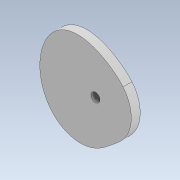
# Autodesk Inventor part: 凸輪
Saved by Autodesk Inventor 2022 (Build 260153000, 153)
## iProperties
Created: 2023-05-12
Part Number: 凸輪
Material: 一般
Document SubType Name: Modeling
Designer: JOU
Density: 1 g/cm^3
Appearance: 預設
Author: JOU
Autodesk Inventor part; units mm, degrees
ref_plane "YZ Plane" through (0, 0, 0) normal (1, 0, 0) x (0, 1, 0)
ref_plane "XZ Plane" through (0, 0, 0) normal (0, 1, 0) x (-1, 0, 0)
ref_plane "XY Plane" through (0, 0, 0) normal (0, 0, 1) x (1, 0, 0)
sketch "草圖1" plane through (0, 0, 0) normal (0, 0, 1) x (1, 0, 0)
  spline S0 degree 3 poles (30.808, 25.5122) (30.6572, 25.6926) (30.3546, 26.0547) (29.8877, 26.5903) (29.4098, 27.1227) (28.9202, 27.6516) (28.4194, 28.177) (27.9076, 28.6992) (27.3849, 29.2182) (26.8516, 29.7342) (26.3079, 30.2472) (25.754, 30.7574) (25.1901, 31.2648) (24.6164, 31.7697) (24.033, 32.2719) (23.44, 32.7717) (22.8377, 33.2691) (22.2261, 33.7641) (21.6054, 34.2567) (20.9756, 34.7471) (20.3368, 35.2351) (19.6892, 35.7208) (19.0327, 36.2041) (18.3675, 36.6849) (17.6935, 37.1633) (17.0109, 37.639) (16.3195, 38.112) (15.6195, 38.5821) (14.9108, 39.0491) (14.1934, 39.5129) (13.4673, 39.9733) (12.7325, 40.4299) (11.9891, 40.8827) (11.2369, 41.3311) (10.4759, 41.775) (9.7063, 42.2141) (8.9279, 42.6479) (8.1408, 43.0762) (7.3451, 43.4985) (6.5407, 43.9144) (5.7276, 44.3234) (4.9061, 44.7252) (4.0761, 45.1193) (3.2377, 45.5052) (2.3911, 45.8823) (1.5363, 46.2503) (0.6736, 46.6085) (-0.1968, 46.9565) (-1.0749, 47.2937) (-1.9604, 47.6195) (-2.853, 47.9335) (-3.7525, 48.2351) (-4.6585, 48.5236) (-5.5709, 48.7987) (-6.4893, 49.0596) (-7.4133, 49.306) (-8.3427, 49.5372) (-9.2769, 49.7527) (-10.2157, 49.9519) (-11.1587, 50.1345) (-12.1054, 50.2998) (-13.0553, 50.4475) (-14.0082, 50.5769) (-14.9634, 50.6877) (-15.9206, 50.7795) (-16.8793, 50.8518) (-17.8389, 50.9042) (-18.7992, 50.9363) (-19.7595, 50.9478) (-20.7194, 50.9384) (-21.6784, 50.9077) (-22.636, 50.8554) (-23.5918, 50.7812) (-24.5453, 50.685) (-25.4959, 50.5664) (-26.4433, 50.4252) (-27.3869, 50.2613) (-28.3262, 50.0745) (-29.2609, 49.8646) (-30.1905, 49.6315) (-31.1144, 49.3752) (-32.0322, 49.0954) (-32.9435, 48.7921) (-33.8478, 48.4653) (-34.7446, 48.115) (-35.6335, 47.7411) (-36.5141, 47.3438) (-37.3858, 46.9229) (-38.2483, 46.4786) (-39.101, 46.011) (-39.9435, 45.5202) (-40.7755, 45.0063) (-41.5963, 44.4694) (-42.4057, 43.9099) (-43.2031, 43.3278) (-43.9881, 42.7235) (-44.7603, 42.0972) (-45.5192, 41.4492) (-46.2646, 40.7799) (-46.9959, 40.0895) (-47.7129, 39.3785) (-48.415, 38.6472) (-49.1021, 37.8962) (-49.7738, 37.1257) (-50.4297, 36.3364) (-51.0696, 35.5287) (-51.6933, 34.703) (-52.3005, 33.86) (-52.8909, 33.0001) (-53.4645, 32.1239) (-54.0211, 31.232) (-54.5605, 30.3248) (-55.0828, 29.4031) (-55.5877, 28.4673) (-56.0753, 27.518) (-56.5456, 26.5558) (-56.9986, 25.5813) (-57.4345, 24.5949) (-57.8531, 23.5973) (-58.2548, 22.589) (-58.6394, 21.5709) (-59.0068, 20.5448) (-59.3563, 19.5118) (-59.6878, 18.473) (-60.0011, 17.4285) (-60.2962, 16.3786) (-60.5728, 15.3238) (-60.831, 14.2644) (-61.0707, 13.2005) (-61.2918, 12.1327) (-61.4942, 11.0612) (-61.6779, 9.9862) (-61.8428, 8.9083) (-61.9888, 7.8276) (-62.116, 6.7446) (-62.2242, 5.6595) (-62.3135, 4.5727) (-62.3839, 3.4844) (-62.4352, 2.3952) (-62.4675, 1.3052) (-62.4807, 0.2148) (-62.475, -0.8757) (-62.4502, -1.9659) (-62.4063, -3.0555) (-62.3435, -4.1442) (-62.2617, -5.2316) (-62.1609, -6.3174) (-62.0412, -7.4013) (-61.9026, -8.483) (-61.7451, -9.562) (-61.5688, -10.6382) (-61.3738, -11.7111) (-61.16, -12.7804) (-60.9277, -13.8459) (-60.6767, -14.9071) (-60.4073, -15.9638) (-60.1195, -17.0156) (-59.8134, -18.0622) (-59.4891, -19.1034) (-59.1466, -20.1387) (-58.7859, -21.1684) (-58.4068, -22.1932) (-58.0082, -23.2137) (-57.5895, -24.2299) (-57.1503, -25.2411) (-56.6899, -26.2468) (-56.2081, -27.2462) (-55.7044, -28.2388) (-55.1784, -29.2238) (-54.6299, -30.2004) (-54.0585, -31.1678) (-53.4641, -32.1253) (-52.8465, -33.072) (-52.2055, -34.007) (-51.5411, -34.9295) (-50.8532, -35.8385) (-50.142, -36.7333) (-49.4074, -37.6127) (-48.6497, -38.4761) (-47.8691, -39.3223) (-47.0658, -40.1505) (-46.2403, -40.9597) (-45.3928, -41.7491) (-44.5238, -42.5176) (-43.634, -43.2645) (-42.7238, -43.9888) (-41.7939, -44.6896) (-40.8451, -45.3662) (-39.878, -46.0177) (-38.8936, -46.6433) (-37.8926, -47.2422) (-36.8761, -47.8139) (-35.845, -48.3575) (-34.8003, -48.8725) (-33.7432, -49.3583) (-32.6746, -49.8144) (-31.5959, -50.2403) (-30.5081, -50.6356) (-29.4126, -51) (-28.3104, -51.3333) (-27.2029, -51.6351) (-26.0914, -51.9054) (-24.9771, -52.1442) (-23.8614, -52.3513) (-22.7454, -52.527) (-21.6306, -52.6714) (-20.5181, -52.7847) (-19.4092, -52.8672) (-18.3052, -52.9193) (-17.2072, -52.9415) (-16.1164, -52.9343) (-15.0339, -52.8983) (-13.9609, -52.8341) (-12.8984, -52.7426) (-11.8473, -52.6245) (-10.8085, -52.4807) (-9.7831, -52.312) (-8.7717, -52.1195) (-7.7752, -51.904) (-6.7942, -51.6668) (-5.8293, -51.4087) (-4.881, -51.131) (-3.9499, -50.8347) (-3.0363, -50.5211) (-2.1405, -50.1911) (-1.2629, -49.8461) (-0.4035, -49.4872) (0.4376, -49.1155) (1.2602, -48.7322) (2.0645, -48.3384) (2.8506, -47.9353) (3.6185, -47.5238) (4.3687, -47.1052) (5.1012, -46.6803) (5.8166, -46.2503) (6.5152, -45.816) (7.1975, -45.3783) (7.8639, -44.9382) (8.515, -44.4964) (9.1514, -44.0537) (9.7737, -43.6107) (10.3826, -43.1681) (10.9787, -42.7265) (11.5627, -42.2865) (12.1353, -41.8484) (12.6974, -41.4126) (13.2495, -40.9796) (13.7925, -40.5495) (14.3271, -40.1225) (14.8541, -39.6988) (15.3742, -39.2785) (15.888, -38.8616) (16.3964, -38.4479) (16.9001, -38.0374) (17.3996, -37.6299) (17.8957, -37.2251) (18.3889, -36.8227) (18.8798, -36.4224) (19.3689, -36.0238) (19.8568, -35.6263) (20.3438, -35.2295) (20.8303, -34.8328) (21.3166, -34.4356) (21.8031, -34.0373) (22.2898, -33.6371) (22.7769, -33.2346) (23.2645, -32.8289) (23.7526, -32.4193) (24.2411, -32.0051) (24.7298, -31.5857) (25.2186, -31.1602) (25.7071, -30.7281) (26.1951, -30.2887) (26.6821, -29.8413) (27.1677, -29.3852) (27.6513, -28.92) (28.1324, -28.4452) (28.6103, -27.9601) (29.0845, -27.4644) (29.5541, -26.9577) (30.018, -26.4402) (30.4743, -25.9129) (30.9219, -25.3771) (31.3601, -24.8336) (31.7887, -24.2825) (32.2077, -23.724) (32.6168, -23.1583) (33.016, -22.5855) (33.4052, -22.0059) (33.7841, -21.4195) (34.1528, -20.8266) (34.5111, -20.2274) (34.8588, -19.622) (35.196, -19.0107) (35.5224, -18.3935) (35.838, -17.7708) (36.1427, -17.1426) (36.4364, -16.5092) (36.7189, -15.8708) (36.9903, -15.2276) (37.2504, -14.5797) (37.4992, -13.9273) (37.7366, -13.2708) (37.9624, -12.6102) (38.1767, -11.9457) (38.3794, -11.2776) (38.5704, -10.6061) (38.7496, -9.9313) (38.917, -9.2535) (39.0726, -8.5729) (39.2163, -7.8897) (39.348, -7.2041) (39.4677, -6.5163) (39.5754, -5.8265) (39.6711, -5.1349) (39.7547, -4.4418) (39.8261, -3.7473) (39.8855, -3.0516) (39.9326, -2.3551) (39.9677, -1.6578) (39.9905, -0.96) (40.0012, -0.2619) (39.9997, 0.4362) (39.9859, 1.1343) (39.9601, 1.8319) (39.922, 2.5291) (39.8718, 3.2254) (39.8094, 3.9208) (39.7349, 4.6149) (39.6483, 5.3077) (39.5497, 5.9989) (39.4389, 6.6882) (39.3162, 7.3755) (39.1815, 8.0605) (39.0349, 8.7431) (38.8763, 9.423) (38.706, 10.1001) (38.5238, 10.774) (38.3299, 11.4447) (38.1243, 12.1119) (37.9071, 12.7755) (37.6784, 13.4351) (37.4382, 14.0906) (37.1866, 14.7418) (36.9236, 15.3886) (36.6494, 16.0307) (36.3641, 16.6678) (36.0676, 17.2999) (35.7602, 17.9268) (35.4419, 18.5481) (35.1128, 19.1639) (34.773, 19.7738) (34.4226, 20.3776) (34.0617, 20.9753) (33.6905, 21.5665) (33.3089, 22.1512) (32.9173, 22.7292) (32.5156, 23.3002) (32.104, 23.8641) (31.6825, 24.4207) (31.2515, 24.971) (30.956, 25.3316) (30.808, 25.5122) knots 0 0 0 0 0.070539 0.141575 0.213119 0.28518 0.357764 0.430881 0.504536 0.578735 0.653483 0.728785 0.804643 0.881062 0.958044 1.035591 1.113703 1.192383 1.271631 1.351446 1.431829 1.51278 1.594297 1.676379 1.759024 1.842232 1.925998 2.010321 2.095198 2.180624 2.266596 2.353108 2.440155 2.527731 2.615827 2.704436 2.793549 2.883156 2.973245 3.063804 3.154819 3.246277 3.338162 3.430457 3.523144 3.616206 3.709622 3.803372 3.897436 3.991791 4.086416 4.181288 4.276384 4.371683 4.46716 4.562793 4.658562 4.754443 4.850417 4.946464 5.042564 5.138701 5.234857 5.33102 5.427174 5.523311 5.619419 5.715491 5.811522 5.907509 6.00345 6.099347 6.195202 6.291021 6.38681 6.482579 6.578338 6.674101 6.769882 6.865697 6.961564 7.057499 7.153524 7.249659 7.345923 7.442339 7.538928 7.635711 7.73271 7.829945 7.927438 8.025206 8.12327 8.221647 8.320354 8.419405 8.518816 8.618599 8.718764 8.819323 8.920283 9.021651 9.123433 9.225633 9.328253 9.431295 9.534758 9.638642 9.742944 9.847661 9.952789 10.058323 10.164258 10.270586 10.377301 10.484395 10.591862 10.699694 10.807881 10.916417 11.025293 11.134336 11.243379 11.352422 11.461465 11.570508 11.679551 11.788595 11.897638 12.006681 12.115724 12.224767 12.33381 12.442854 12.551897 12.66094 12.769983 12.879026 12.988069 13.097113 13.206156 13.315199 13.424242 13.533285 13.642328 13.751372 13.860415 13.969458 14.078501 14.187544 14.296587 14.405631 14.514674 14.623717 14.73276 14.841803 14.950846 15.059889 15.168933 15.277976 15.387019 15.496229 15.605779 15.715673 15.825915 15.936509 16.047456 16.158756 16.270409 16.382411 16.494759 16.607449 16.720476 16.833833 16.94751 17.0615 17.175792 17.290375 17.405234 17.520356 17.635725 17.751323 17.867133 17.983134 18.099303 18.215619 18.332055 18.448587 18.565185 18.681821 18.798464 18.915083 19.031643 19.148112 19.264453 19.380629 19.496605 19.612341 19.7278 19.842942 19.957728 20.072119 20.186074 20.299556 20.412523 20.524938 20.636761 20.747954 20.85848 20.968301 21.077381 21.185685 21.293177 21.399825 21.505595 21.610456 21.714377 21.817329 21.919284 22.020214 22.120094 22.218901 22.316611 22.413204 22.50866 22.602963 22.696096 22.788045 22.878799 22.968348 23.056685 23.143806 23.229706 23.314387 23.397851 23.480103 23.561152 23.641009 23.719687 23.797205 23.873583 23.948844 24.023016 24.096129 24.168219 24.239321 24.309477 24.378731 24.447132 24.514729 24.581578 24.647734 24.713258 24.77821 24.842656 24.90666 24.970288 25.033609 25.096688 25.159594 25.222391 25.285146 25.347919 25.410771 25.47376 25.536938 25.600355 25.664058 25.728087 25.79248 25.85727 25.922483 25.988145 26.054272 26.12088 26.187979 26.255575 26.323671 26.392264 26.461351 26.530924 26.600736 26.670548 26.740361 26.810173 26.879985 26.949798 27.01961 27.089422 27.159234 27.229047 27.298859 27.368671 27.438484 27.508296 27.578108 27.64792 27.717733 27.787545 27.857357 27.92717 27.996982 28.066794 28.136606 28.206419 28.276231 28.346043 28.415856 28.485668 28.55548 28.625292 28.695105 28.764917 28.834729 28.904542 28.974354 29.044166 29.113978 29.183791 29.253603 29.323415 29.393228 29.46304 29.532852 29.602664 29.672477 29.742289 29.812101 29.881914 29.951726 30.021538 30.09135 30.161163 30.230975 30.300787 30.3706 30.440412 30.510224 30.580036 30.649849 30.719661 30.789473 30.859286 30.929098 30.99891 31.068722 31.138535 31.208347 31.278159 31.347971 31.417784 31.487596 31.557408 31.627221 31.697033 31.766845 31.836658 31.90647 31.976282 32.046094 32.115907 32.185959 32.185959 32.185959 32.185959
  circle A0 centre (0, 0) radius 5
  point P0 (29.8876, 26.5879)
  point P1 (29.4096, 27.1202)
  point P2 (28.9202, 27.6491)
  point P3 (28.4194, 28.1746)
  point P4 (27.9077, 28.6968)
  point P5 (27.3851, 29.2158)
  point P6 (26.8519, 29.7318)
  point P7 (26.3082, 30.2448)
  point P8 (25.7544, 30.7551)
  point P9 (25.1906, 31.2625)
  point P10 (24.6169, 31.7674)
  point P11 (24.0335, 32.2697)
  point P12 (23.4406, 32.7695)
  point P13 (22.8383, 33.2669)
  point P14 (22.2268, 33.7619)
  point P15 (21.6061, 34.2546)
  point P16 (20.9763, 34.745)
  point P17 (20.3376, 35.233)
  point P18 (19.69, 35.7187)
  point P19 (19.0335, 36.202)
  point P20 (18.3683, 36.6829)
  point P21 (17.6944, 37.1612)
  point P22 (17.0117, 37.637)
  point P23 (16.3204, 38.1099)
  point P24 (15.6203, 38.5801)
  point P25 (14.9116, 39.0471)
  point P26 (14.1942, 39.5109)
  point P27 (13.4682, 39.9712)
  point P28 (12.7334, 40.4279)
  point P29 (11.9899, 40.8806)
  point P30 (11.2377, 41.329)
  point P31 (10.4767, 41.7729)
  point P32 (9.707, 42.212)
  point P33 (8.9286, 42.6458)
  point P34 (8.1415, 43.0741)
  point P35 (7.3457, 43.4963)
  point P36 (6.5413, 43.9122)
  point P37 (5.7282, 44.3212)
  point P38 (4.9066, 44.723)
  point P39 (4.0765, 45.1171)
  point P40 (3.2381, 45.5029)
  point P41 (2.3914, 45.88)
  point P42 (1.5366, 46.248)
  point P43 (0.6739, 46.6062)
  point P44 (-0.1967, 46.9541)
  point P45 (-1.0748, 47.2913)
  point P46 (-1.9603, 47.6171)
  point P47 (-2.853, 47.931)
  point P48 (-3.7525, 48.2326)
  point P49 (-4.6586, 48.5211)
  point P50 (-5.5711, 48.7961)
  point P51 (-6.4895, 49.057)
  point P52 (-7.4136, 49.3033)
  point P53 (-8.3429, 49.5344)
  point P54 (-9.2772, 49.7499)
  point P55 (-10.2161, 49.9491)
  point P56 (-11.159, 50.1316)
  point P57 (-12.1057, 50.2968)
  point P58 (-13.0557, 50.4444)
  point P59 (-14.0085, 50.5738)
  point P60 (-14.9638, 50.6846)
  point P61 (-15.9209, 50.7763)
  point P62 (-16.8796, 50.8485)
  point P63 (-17.8392, 50.9008)
  point P64 (-18.7994, 50.9329)
  point P65 (-19.7596, 50.9443)
  point P66 (-20.7195, 50.9348)
  point P67 (-21.6784, 50.9041)
  point P68 (-22.6359, 50.8517)
  point P69 (-23.5916, 50.7775)
  point P70 (-24.5449, 50.6812)
  point P71 (-25.4955, 50.5626)
  point P72 (-26.4427, 50.4214)
  point P73 (-27.3861, 50.2575)
  point P74 (-28.3254, 50.0707)
  point P75 (-29.2599, 49.8608)
  point P76 (-30.1893, 49.6277)
  point P77 (-31.113, 49.3713)
  point P78 (-32.0307, 49.0916)
  point P79 (-32.9418, 48.7884)
  point P80 (-33.8459, 48.4616)
  point P81 (-34.7426, 48.1114)
  point P82 (-35.6313, 47.7376)
  point P83 (-36.5117, 47.3403)
  point P84 (-37.3833, 46.9195)
  point P85 (-38.2456, 46.4753)
  point P86 (-39.0982, 46.0078)
  point P87 (-39.9406, 45.517)
  point P88 (-40.7724, 45.0032)
  point P89 (-41.5931, 44.4665)
  point P90 (-42.4023, 43.9071)
  point P91 (-43.1996, 43.3252)
  point P92 (-43.9845, 42.721)
  point P93 (-44.7566, 42.0948)
  point P94 (-45.5155, 41.4469)
  point P95 (-46.2608, 40.7777)
  point P96 (-46.9921, 40.0875)
  point P97 (-47.709, 39.3766)
  point P98 (-48.4111, 38.6454)
  point P99 (-49.0982, 37.8945)
  point P100 (-49.7698, 37.1242)
  point P101 (-50.4257, 36.335)
  point P102 (-51.0656, 35.5273)
  point P103 (-51.6893, 34.7018)
  point P104 (-52.2965, 33.8589)
  point P105 (-52.887, 32.9991)
  point P106 (-53.4606, 32.123)
  point P107 (-54.0172, 31.2312)
  point P108 (-54.5567, 30.3241)
  point P109 (-55.0789, 29.4025)
  point P110 (-55.5839, 28.4668)
  point P111 (-56.0716, 27.5176)
  point P112 (-56.5419, 26.5554)
  point P113 (-56.995, 25.5809)
  point P114 (-57.4309, 24.5947)
  point P115 (-57.8497, 23.5971)
  point P116 (-58.2514, 22.5888)
  point P117 (-58.6362, 21.5704)
  point P118 (-59.0038, 20.5437)
  point P119 (-59.3533, 19.5109)
  point P120 (-59.6848, 18.472)
  point P121 (-59.9981, 17.4276)
  point P122 (-60.2931, 16.3778)
  point P123 (-60.5698, 15.3231)
  point P124 (-60.828, 14.2636)
  point P125 (-61.0676, 13.1999)
  point P126 (-61.2887, 12.1321)
  point P127 (-61.4911, 11.0606)
  point P128 (-61.6748, 9.9857)
  point P129 (-61.8396, 8.9078)
  point P130 (-61.9857, 7.8272)
  point P131 (-62.1128, 6.7442)
  point P132 (-62.2211, 5.6592)
  point P133 (-62.3104, 4.5724)
  point P134 (-62.3807, 3.4843)
  point P135 (-62.432, 2.395)
  point P136 (-62.4643, 1.3051)
  point P137 (-62.4776, 0.2147)
  point P138 (-62.4718, -0.8757)
  point P139 (-62.447, -1.9658)
  point P140 (-62.4032, -3.0554)
  point P141 (-62.3403, -4.144)
  point P142 (-62.2585, -5.2314)
  point P143 (-62.1577, -6.3171)
  point P144 (-62.038, -7.401)
  point P145 (-61.8994, -8.4825)
  point P146 (-61.7419, -9.5615)
  point P147 (-61.5657, -10.6376)
  point P148 (-61.3706, -11.7105)
  point P149 (-61.1569, -12.7798)
  point P150 (-60.9246, -13.8452)
  point P151 (-60.6737, -14.9063)
  point P152 (-60.4043, -15.963)
  point P153 (-60.1165, -17.0147)
  point P154 (-59.8104, -18.0613)
  point P155 (-59.486, -19.1024)
  point P156 (-59.1436, -20.1377)
  point P157 (-58.7831, -21.1668)
  point P158 (-58.4041, -22.191)
  point P159 (-58.0055, -23.2114)
  point P160 (-57.5868, -24.2275)
  point P161 (-57.1475, -25.2386)
  point P162 (-56.6871, -26.2441)
  point P163 (-56.2052, -27.2435)
  point P164 (-55.7015, -28.236)
  point P165 (-55.1755, -29.2208)
  point P166 (-54.627, -30.1973)
  point P167 (-54.0556, -31.1647)
  point P168 (-53.4612, -32.1221)
  point P169 (-52.8435, -33.0686)
  point P170 (-52.2025, -34.0036)
  point P171 (-51.5381, -34.926)
  point P172 (-50.8503, -35.8349)
  point P173 (-50.139, -36.7296)
  point P174 (-49.4045, -37.609)
  point P175 (-48.6468, -38.4722)
  point P176 (-47.8662, -39.3184)
  point P177 (-47.0629, -40.1465)
  point P178 (-46.2374, -40.9557)
  point P179 (-45.3899, -41.745)
  point P180 (-44.521, -42.5135)
  point P181 (-43.6311, -43.2603)
  point P182 (-42.721, -43.9845)
  point P183 (-41.7911, -44.6853)
  point P184 (-40.8423, -45.3618)
  point P185 (-39.8753, -46.0133)
  point P186 (-38.8908, -46.6388)
  point P187 (-37.8899, -47.2377)
  point P188 (-36.8734, -47.8093)
  point P189 (-35.8423, -48.3529)
  point P190 (-34.7977, -48.8679)
  point P191 (-33.7405, -49.3537)
  point P192 (-32.672, -49.8097)
  point P193 (-31.5933, -50.2356)
  point P194 (-30.5055, -50.6309)
  point P195 (-29.41, -50.9953)
  point P196 (-28.3078, -51.3285)
  point P197 (-27.2003, -51.6303)
  point P198 (-26.0888, -51.9006)
  point P199 (-24.9745, -52.1394)
  dimension "d0" = 10
  constraints: 1 centre point, 1 coincident, 360 other
  measures "d0" diameter of A0
extrude "擠出1" add sketch "草圖1" along normal blind 10
